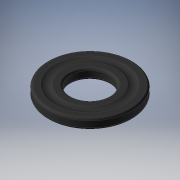
# Autodesk Inventor part: 51200 Housing washer
Saved by Autodesk Inventor 2019 (Build 230136000, 136)
## iProperties
Created: 2023-01-10
Part Number: 51200 Housing washer
Material: Generic
Catalog Web Link: www.cadenas.de
Description: With flat seet HW-
Vendor: NSK_RB
Document SubType Name: Modeling
Designer: psAdmin
Manufacturer: NSK_RB
Mass: 1.22727 g
Surface Area: 11.4478 cm^2
Volume: 1.22727 cm^3
Density: 1 g/cm^3
Appearance: PSOLRGB-175-175-175
Category: PARTsolutions
Company: NSK_RB
Title: 51200 Housing washer
Author: Cadenas PARTsolutions
PSOL_IDENT_0: {$CADENAS_DATA/23d-libs/nsk_rb/roller_bearings/thrust_bearings/single_direction_tbb/with_flat_seet_h
PSOL_IDENT_1: w.prj},193 {VTYP=3D},{NB=51200 Housing washer},{LINA=51200 Housing washer},{NN=With flat seet HW},{D
PSOL_IDENT_2: ATE=27.09.2022 23:23:10},{GEOMDATE=23.08.2022 10:33:13},{VERSION=},{LINEID=6260},{WBVAR=},{WBNUMERIC=
PSOL_IDENT_3: }  {NB=51200 Housing washer},{LINA=51200 Housing washer},{KT=DUMMY},{N=10},{IDNR=},{STAN=},{NO=2},{O
PSOL_IDENT_4: RDER=51200},{SD=10},{D=26},{T=11},{T3=11.6},{T4=13},{SR=0.6},{CAN=12800},{COAN=17100},{CA=1300},{COA=
PSOL_IDENT_5: 1740},{GRE=6000},{OIL=9000},{SD1=26},{D1=12},{D2=18},{D3=28},{SB=3.5},{A=8.5},{R=22},{SDA=20},{DA=16
PSOL_IDENT_6: },{SRA=0.6},{MASS=0.028},{DIST=1.233}
NB: 51200 Housing washer
NN: With flat seet HW
NBSYN: $ORDER. Housing washer
LINA: 51200 Housing washer
CATALOG: NSK Rolling Bearing
N: 10
NO: 2
ORDER: 51200
SD: 10
D: 26
T: 11
T3: 11.6
T4: 13
SR: 0.6
CAN: 12800
COAN: 17100
CA: 1300
COA: 1740
GRE: 6000
OIL: 9000
SD1: 26
D1: 12
D2: 18
D3: 28
SB: 3.5
A: 8.5
R: 22
SDA: 20
DA: 16
SRA: 0.6
MASS: 0.028
SUPPLIER: NSK_RB
ARTICLENO: 51200 Housing washer
BOMINFO: 51200 Housing washer
CREATOR: CADENAS GmbH
Autodesk Inventor part; units mm, degrees
sketch "Sketch_1" plane through (0, 0, 0) normal (0, 0, 1) x (0, 1, 0)
  line L0 (3.0556, 0) -> (0, 0)
  arc A0 (0, 6.6) -> (0.6, 6) centre (0.6, 6.6) ccw
  line L1 (0.6, 6) -> (2.4556, 6)
  arc A1 (2.4556, 6) -> (3.0556, 6.6) centre (2.4556, 6.6) ccw
  line L2 (3.0556, 6.6) -> (3.0556, 8.2402)
  arc A2 (3.0556, 10.7598) -> (3.0556, 8.2402) centre (5.5, 9.5) ccw
  line L3 (3.0556, 10.7598) -> (3.0556, 12.4)
  arc A3 (3.0556, 12.4) -> (2.4556, 13) centre (2.4556, 12.4) ccw
  line L4 (2.4556, 13) -> (0.6, 13)
  arc A4 (0.6, 13) -> (0, 12.4) centre (0.6, 12.4) ccw
  line L5 (0, 12.4) -> (0, 6.6)
  constraints: 12 end point, 10 point on circle, 5 centre point
revolve "Revolution1" add sketch "Sketch_1" angle 360 about axis through (0, 3.0556, 0) along (0, 1, 0)
ref_plane "HW_B_1_XY" through (-9.5, 5.5, 0) normal (0, 1, 0) x (0, 0, -1)
ref_plane "HW_B_1_YZ" through (-9.5, 5.5, 0) normal (0, 0, -1) x (-1, 0, 0)
ref_plane "HW_B_1_ZX" through (-9.5, 5.5, 0) normal (-1, 0, 0) x (0, 1, 0)
ref_plane "HW_B_10_XY" through (-7.6857, 5.5, -5.584) normal (0, 1, 0) x (0, 0, -1)
ref_plane "HW_B_10_YZ" through (-7.6857, 5.5, -5.584) normal (0, 0, -1) x (-1, 0, 0)
ref_plane "HW_B_10_ZX" through (-7.6857, 5.5, -5.584) normal (-1, 0, 0) x (0, 1, 0)
ref_plane "HW_B_2_XY" through (-7.6857, 5.5, 5.584) normal (0, 1, 0) x (0, 0, -1)
ref_plane "HW_B_2_YZ" through (-7.6857, 5.5, 5.584) normal (0, 0, -1) x (-1, 0, 0)
ref_plane "HW_B_2_ZX" through (-7.6857, 5.5, 5.584) normal (-1, 0, 0) x (0, 1, 0)
ref_plane "HW_B_3_XY" through (-2.9357, 5.5, 9.035) normal (0, 1, 0) x (0, 0, -1)
ref_plane "HW_B_3_YZ" through (-2.9357, 5.5, 9.035) normal (0, 0, -1) x (-1, 0, 0)
ref_plane "HW_B_3_ZX" through (-2.9357, 5.5, 9.035) normal (-1, 0, 0) x (0, 1, 0)
ref_plane "HW_B_4_XY" through (2.9357, 5.5, 9.035) normal (0, 1, 0) x (0, 0, -1)
ref_plane "HW_B_4_YZ" through (2.9357, 5.5, 9.035) normal (0, 0, -1) x (-1, 0, 0)
ref_plane "HW_B_4_ZX" through (2.9357, 5.5, 9.035) normal (-1, 0, 0) x (0, 1, 0)
ref_plane "HW_B_5_XY" through (7.6857, 5.5, 5.584) normal (0, 1, 0) x (0, 0, -1)
ref_plane "HW_B_5_YZ" through (7.6857, 5.5, 5.584) normal (0, 0, -1) x (-1, 0, 0)
ref_plane "HW_B_5_ZX" through (7.6857, 5.5, 5.584) normal (-1, 0, 0) x (0, 1, 0)
ref_plane "HW_B_6_XY" through (9.5, 5.5, 0) normal (0, 1, 0) x (0, 0, -1)
ref_plane "HW_B_6_YZ" through (9.5, 5.5, 0) normal (0, 0, -1) x (-1, 0, 0)
ref_plane "HW_B_6_ZX" through (9.5, 5.5, 0) normal (-1, 0, 0) x (0, 1, 0)
ref_plane "HW_B_7_XY" through (7.6857, 5.5, -5.584) normal (0, 1, 0) x (0, 0, -1)
ref_plane "HW_B_7_YZ" through (7.6857, 5.5, -5.584) normal (0, 0, -1) x (-1, 0, 0)
ref_plane "HW_B_7_ZX" through (7.6857, 5.5, -5.584) normal (-1, 0, 0) x (0, 1, 0)
ref_plane "HW_B_8_XY" through (2.9357, 5.5, -9.035) normal (0, 1, 0) x (0, 0, -1)
ref_plane "HW_B_8_YZ" through (2.9357, 5.5, -9.035) normal (0, 0, -1) x (-1, 0, 0)
ref_plane "HW_B_8_ZX" through (2.9357, 5.5, -9.035) normal (-1, 0, 0) x (0, 1, 0)
ref_plane "HW_B_9_XY" through (-2.9357, 5.5, -9.035) normal (0, 1, 0) x (0, 0, -1)
ref_plane "HW_B_9_YZ" through (-2.9357, 5.5, -9.035) normal (0, 0, -1) x (-1, 0, 0)
ref_plane "HW_B_9_ZX" through (-2.9357, 5.5, -9.035) normal (-1, 0, 0) x (0, 1, 0)
ref_plane "HW_SW_XY" through (0, 0, 0) normal (0, 1, 0) x (0, 0, -1)
ref_plane "HW_SW_YZ" through (0, 0, 0) normal (0, 0, -1) x (-1, 0, 0)
ref_plane "HW_SW_ZX" through (0, 0, 0) normal (-1, 0, 0) x (0, 1, 0)
body "Solid1"
